DHEC proto sensor v2 (Autodesk Fusion 360 design; units mm, degrees)
Autodesk Fusion 360 part; units mm, degrees
note: some values were not read from the file. Set by a fixed rule: which sketch regions a step uses.
sketch "Sketch1" plane through (0, 0, 0) normal (0, 0, 1) x (1, 0, 0)
  circle A0 centre (0, 0) radius 38.1
  circle A1 centre (0, 0) radius 36.1
  line L0 (23.3872, -27.5) -> (23.3872, 27.5)
  line L1 (25.3872, -25.6652) -> (25.3872, 25.6652)
  line L2 (25.3872, 12.5) -> (27.3872, 12.5)
  line L3 (27.3872, 12.5) -> (27.3872, -12.5)
  line L4 (27.3872, -12.5) -> (25.3872, -12.5)
  line L5 (25.3872, -12.5) -> (25.3872, 12.5)
  line L6 (25.3872, 14.5) -> (29.3872, 14.5)
  line L7 (29.3872, 14.5) -> (29.3872, 9.5)
  line L8 (29.3872, 9.5) -> (27.3872, 9.5)
  line L9 (25.3872, -14.5) -> (29.3872, -14.5)
  line L10 (29.3872, -14.5) -> (29.3872, -9.5)
  line L11 (29.3872, -9.5) -> (27.3872, -9.5)
  line L12 (1.75, 0) -> (22.5, 0)
  line L13 (23.3872, 26.75) -> (20.8872, 26.75)
  line L14 (20.8872, 26.75) -> (20.8872, -26.75)
  line L15 (20.8872, -26.75) -> (23.3872, -26.75)
  line L16 (23.3872, -26.75) -> (23.3872, 26.75)
  line L17 (20.8872, 18.08) -> (8.8872, 18.08)
  line L18 (8.8872, 18.08) -> (8.8872, 5.08)
  line L19 (8.8872, 5.08) -> (20.8872, 5.08)
  line L20 (20.8872, 5.08) -> (20.8872, 18.08)
  line L21 (20.8872, -12.5) -> (8.8872, -12.5)
  line L22 (8.8872, -12.5) -> (8.8872, -22.5)
  line L23 (8.8872, -22.5) -> (20.8872, -22.5)
  line L24 (20.8872, -22.5) -> (20.8872, -12.5)
  line L25 (29.3872, -9.5) -> (29.3872, 9.5)
  line L26 (0, -38.1) -> (0, 38.1) construction
  line L27 (-38.1, 0) -> (38.1, 0) construction
  line L28 (26.9408, -26.9408) -> (-26.9408, 26.9408) construction
  line L29 (26.9408, 26.9408) -> (-26.9408, -26.9408) construction
  line L30 (0, 36.1) -> (0, 38.1)
  line L31 (-25.5266, 25.5266) -> (-26.9408, 26.9408)
  line L32 (-36.1, 0) -> (-38.1, 0)
  line L33 (-26.9408, -26.9408) -> (-25.5266, -25.5266)
  line L34 (0, -38.1) -> (0, -36.1)
  line L35 (26.9408, -26.9408) -> (25.5266, -25.5266)
  line L36 (38.1, 0) -> (36.1, 0)
  line L37 (26.9408, 26.9408) -> (25.5266, 25.5266)
  line L38 (18.8872, 30.765) -> (18.8872, 20.08)
  line L39 (18.8872, 20.08) -> (6.8872, 20.08)
  line L40 (6.8872, 20.08) -> (6.8872, 3.08)
  line L41 (6.8872, 3.08) -> (20.8872, 3.08)
  line L42 (-37.7705, 5) -> (-35.7705, 5)
  line L43 (-35.7705, 5) -> (-35.7705, -5)
  line L44 (-35.7705, -5) -> (-37.7705, -5)
  line L45 (-37.7705, -5) -> (-37.7705, 5)
  line L46 (-12.7705, 5) -> (-10.7705, 5)
  line L47 (-10.7705, 5) -> (-10.7705, -5)
  line L48 (-10.7705, -5) -> (-12.7705, -5)
  line L49 (-12.7705, -5) -> (-12.7705, 5)
  line L50 (-29.2705, 24) -> (-19.2705, 24)
  line L51 (-19.2705, 24) -> (-19.2705, 22)
  line L52 (-19.2705, 22) -> (-29.2705, 22)
  line L53 (-29.2705, 22) -> (-29.2705, 24)
  line L54 (-29.2705, -22) -> (-19.2705, -22)
  line L55 (-19.2705, -22) -> (-19.2705, -24)
  line L56 (-19.2705, -24) -> (-29.2705, -24)
  line L57 (-29.2705, -24) -> (-29.2705, -22)
  line L58 (-25.7705, 16.5) -> (-17.7705, 16.5)
  line L59 (-17.7705, 16.5) -> (-17.7705, 0.5)
  line L60 (-17.7705, 0.5) -> (-25.7705, 0.5)
  line L61 (-25.7705, 0.5) -> (-25.7705, 16.5)
  point P0 (27.3872, 0)
  point P1 (20.8872, 0)
  point P2 (-33.5, 0)
  point P3 (-20, 24)
  point P4 (-35.7705, 0)
  point P5 (-24.2705, 0)
  point P6 (-24.2705, 22)
  dimension "d1" = 76.2
  dimension "d2" = 2
  dimension "d3" = 55
  dimension "d4" = 2
  dimension "d5" = 2
  dimension "d6" = 2
  dimension "d7" = 2
  dimension "d8" = 3
  dimension "d9" = 25
  dimension "d10" = 2
  dimension "d11" = 2.5
  dimension "d12" = 53.5
  dimension "d13" = 13
  dimension "d14" = 12
  dimension "d15" = 8.67
  dimension "d16" = 10
  dimension "d17" = 12
  dimension "d18" = 4.25
  dimension "d23" = 45
  dimension "d27" = 2
  dimension "d28" = 2
  dimension "d29" = 2
  dimension "d30" = 2
  dimension "d45" = 10
  dimension "d46" = 2
  dimension "d47" = 11.5
  dimension "d48" = 11.5
  dimension "d49" = 22
  dimension "d50" = 22
  dimension "d51" = 16
  dimension "d52" = 8
  dimension "d53" = 1.5
  dimension "d54" = 5.5
  constraint coincident A0.centre A1.centre
  constraint coincident A1 L0.start
  constraint coincident A1 L0.end
  constraint vertical L0
  constraint coincident A1 L1.start
  constraint coincident A1 L1.end
  constraint parallel L0 L1
  constraint horizontal L2
  constraint vertical L3
  constraint horizontal L4
  constraint vertical L5
  constraint coincident L1 L2.start
  constraint coincident L1 L6.start
  constraint perpendicular L1 L6
  constraint perpendicular L6 L7
  constraint coincident L3 L8.end
  constraint perpendicular L3 L8
  constraint coincident L1 L9.start
  constraint perpendicular L1 L9
  constraint perpendicular L9 L10
  constraint coincident L3 L11.end
  constraint perpendicular L3 L11
  constraint equal L6 L9
  constraint equal L7 L10
  constraint midpoint L3 P0
  constraint coincident P0 L12
  constraint horizontal L13
  constraint vertical L14
  constraint horizontal L15
  constraint vertical L16
  constraint coincident L0 L13.start
  constraint midpoint L14 P1
  constraint coincident L12 P1
  constraint horizontal L17
  constraint vertical L18
  constraint horizontal L19
  constraint vertical L20
  constraint coincident L14 L17.start
  constraint horizontal L21
  constraint vertical L22
  constraint horizontal L23
  constraint vertical L24
  constraint coincident L14 L21.start
  constraint coincident A0 L26.start
  constraint coincident A0 L26.end
  constraint vertical L26
  constraint coincident A0 L27.start
  constraint coincident A0 L27.end
  constraint perpendicular L3 L27
  constraint coincident A0 L28.start
  constraint coincident A0 L28.end
  constraint coincident A0 L29.start
  constraint coincident A0 L29.end
  constraint coincident A0.centre L29
  constraint coincident A0.centre L28
  constraint coincident A0.centre L26
  constraint coincident A0.centre L27
  constraint perpendicular L28 L29
  constraint coincident L26 L30.start
  constraint coincident A1 L30.start
  constraint coincident A1 L31.start
  constraint coincident L28 L31.start
  constraint coincident A1 L32.start
  constraint coincident L27 L32.start
  constraint coincident L29 L33.end
  constraint coincident A1 L33.end
  constraint coincident A1 L34.end
  constraint coincident L26 L34.end
  constraint coincident L28 L35.end
  constraint coincident A1 L35.end
  constraint coincident A1 L36.end
  constraint coincident L27 L36.end
  constraint coincident A1 L37.end
  constraint coincident L29 L37.end
  constraint perpendicular L38 L39
  constraint coincident L14 L41.end
  constraint perpendicular L14 L41
  constraint coincident A1 L38.start
  constraint coincident L27 P2
  constraint horizontal L42
  constraint vertical L43
  constraint horizontal L44
  constraint vertical L45
  constraint horizontal L46
  constraint vertical L47
  constraint horizontal L48
  constraint vertical L49
  constraint horizontal L50
  constraint vertical L51
  constraint horizontal L52
  constraint vertical L53
  constraint horizontal L54
  constraint vertical L55
  constraint horizontal L56
  constraint vertical L57
  constraint equal L45 L50
  constraint equal L47 L50
  constraint equal L50 L54
  constraint midpoint L43 P4
  constraint coincident L27 P4
  constraint coincident L42.end L46
  constraint coincident A0 L42.start
  constraint equal L42 L51
  constraint coincident L27 P5
  constraint midpoint L52 P6
  constraint vertical P5 P6
  constraint coincident L51.end L55
  constraint equal L51 L55
  constraint equal L46 L51
  constraint horizontal L58
  constraint vertical L59
  constraint horizontal L60
  constraint vertical L61
  measures "d1" diameter of A0
  measures "d2" distance of A0 A1
  measures "d3" distance of L0.start L0.end
  measures "d4" distance of L0 L1
  measures "d5" distance of L3 L5
  measures "d6" distance of L4 L9
  measures "d7" distance of L3 L10
  measures "d8" distance of L4 L11
  measures "d9" distance of L2 L4
  measures "d10" distance of L2 L6
  measures "d11" distance of L0 L14
  measures "d12" distance of L13.end L14.end
  measures "d13" distance of L17 L19
  measures "d14" distance of L18 L20
  measures "d15" distance of L13.end L17
  measures "d16" distance of L21 L23
  measures "d17" distance of L14 L22
  measures "d18" distance of L15 L23
  measures "d23" angle of L27 L28
  measures "d27" distance of L18 L40
  measures "d28" distance of L17 L39
  measures "d29" distance of L19 L41
  measures "d30" distance of L14 L38
  measures "d45" distance of L50.start L50.end
  measures "d46" distance of L50 L52
  measures "d47" distance of L43 P5
  measures "d48" distance of L49 P5
  measures "d49" distance of L27 L52
  measures "d50" distance of L54 P5
  measures "d51" distance of L58 L60
  measures "d52" distance of L59 L61
  measures "d53" distance of P6 L61
  measures "d54" distance of L52 L58
extrude "Extrude1" add sketch "Sketch1" along normal blind 2 contours A0 A1 L36 L37 | A0 A1 L35 L36 | A0 A1 L30 L37 | A0 A1 L34 L35 | A1 L1 L6 L7 L9 L10 L25 | A0 A1 L30 L31 | A0 A1 L33 L34 | A0 A1 L31 L42 L43 L50 L52 L53 | A1 L0 L14 L15 L21 L22 L23 L38 L39 L40 L41 L43 L50 L51 L52 L54 L55 L56 | A0 A1 L33 L43 L44 L54 L56 L57 | A0 L32 L45 | A1 L32 L42 L43 L45 | A1 L0 L13 L14 L17 L18 L19 L38 L39 L40 L41 | A1 L32 L43 L44 L45 | A0 L32 L45 | A1 L50 L51 L52 | A1 L50 L52 L53 | L0 L13 L14 L15 L16 L20 L24 | A1 L54 L56 L57 | A1 L54 L55 L56 | A1 L43 | L46 L47 L48 L49
extrude "Extrude4" add sketch "Sketch1" along normal blind 10 contours A1 L0 L13 L14 L17 L18 L19 L38 L39 L40 L41
extrude "Extrude6" add sketch "Sketch1" along normal blind 50 contours A1 L0 L1 L5 L16
extrude "Extrude7" add sketch "Sketch1" along normal blind 15 contours A1 L32 L42 L43 L45 | L1 L2 L3 L6 L7 L8 | A1 L32 L43 L44 L45 | L1 L3 L4 L9 L10 L11 | A1 L50 L51 L52 | A1 L50 L52 L53 | A1 L54 L56 L57 | A1 L54 L55 L56 | A1 L43 | L46 L47 L48 L49
equation "d47 = ( 23 / 2 ) * 1 mm"
